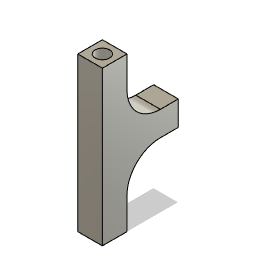
JOINTO v3 (Autodesk Fusion 360 design; units mm, degrees)
Autodesk Fusion 360 part; units mm, degrees
sketch "スケッチ2" plane through (0, 0, 0) normal (0, 1, 0) x (1, 0, 0)
  circle A0 centre (0, 0) radius 1.4
  circle A1 centre (0, 0) radius 2.4
  line L0 (2.4, -2.4) -> (-2.4, -2.4)
  line L1 (-2.4, -2.4) -> (-2.4, 2.4)
  line L2 (-2.4, 2.4) -> (2.4, 2.4)
  line L3 (2.4, 2.4) -> (2.4, -2.4)
  dimension "d1" = 2.8
  dimension "d2" = 1
  constraint coincident A0.centre A1.centre
  constraint horizontal L0
  constraint vertical L1
  constraint horizontal L2
  constraint vertical L3
  constraint tangent A1 L0
  constraint tangent A1 L3
  constraint tangent A1 L2
  constraint tangent A1 L1
  measures "d1" diameter of A0
extrude "押し出し1" add sketch "スケッチ2" along normal blind 30
sketch "スケッチ3" plane through (0, 0, -2.4) normal (0, 0, -1) x (-1, 0, 0)
  circle A0 centre (0, 15) radius 1.4
  circle A1 centre (0, 15) radius 2.4
  line L0 (0, 30) -> (0, 0) construction
  line L1 (2.25, 30) -> (-2.25, 30) construction
  line L2 (-2.4, 0) -> (2.4, 0)
  line L3 (2.4, 0) -> (2.4, 30)
  line L4 (2.4, 30) -> (-2.4, 30)
  line L5 (-2.4, 30) -> (-2.4, 0)
  line L6 (2.4, 12.6) -> (-2.4, 12.6)
  line L7 (-2.4, 12.6) -> (-2.4, 17.4)
  line L8 (-2.4, 17.4) -> (2.4, 17.4)
  line L9 (2.4, 17.4) -> (2.4, 12.6)
  dimension "d6" = 2.8
  dimension "d7" = 1
  constraint coincident L0.end origin
  constraint vertical L0
  constraint midpoint A0.centre L0
  constraint coincident L0.start L1
  constraint horizontal L6
  constraint vertical L7
  constraint horizontal L8
  constraint vertical L9
  constraint coincident L3 L6.start
  constraint tangent A1 L8
  constraint tangent A1 L7
  constraint tangent A1 L6
  measures "d6" diameter of A0
extrude "押し出し2" add sketch "スケッチ3" along normal blind 10 contours A1 | A1 L3 L6 L9 | A1 L3 L8 L9 | A1 L5 L7 L8 | A1 L5 L6 L7
fillet "フィレット1" radius 6.5 1 edges at (0, 12.6, -2.4)
fillet "フィレット2" radius 6.5 1 edges at (0, 17.4, -2.4)
